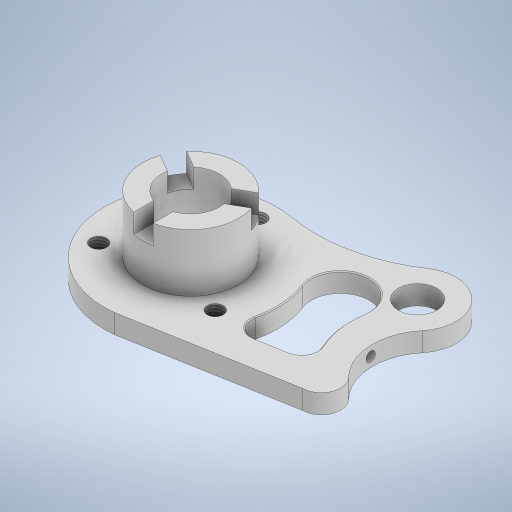
# Autodesk Inventor part: Curved disk example
Saved by Autodesk Inventor 2024 (Build 280153000, 153)
## iProperties
Created: 2023-05-09
Part Number: Curved disk example
Material: Generic
Document SubType Name: Modeling
Designer: Raj
Density: 1 g/cm^3
Appearance: Default
Author: Raj
Autodesk Inventor part; units mm, degrees
ref_plane "YZ Plane" through (0, 0, 0) normal (1, 0, 0) x (0, 1, 0)
ref_plane "XZ Plane" through (0, 0, 0) normal (0, 1, 0) x (-1, 0, 0)
sketch "Sketch1" plane through (0, 0, 0) normal (0, 0, 1) x (1, 0, 0)
  arc A0 (93.3944, 27.2324) -> (66.8467, 56.6014) centre (78, 40) ccw
  circle A1 centre (78, 40) radius 10
  arc A2 (88.012, -30) -> (95.1215, -12.9797) centre (88, -20) ccw
  arc A3 (93.3944, 27.2324) -> (95.1215, -12.9797) centre (116.4861, 8.081) ccw
  arc A4 (70.653, 19.7601) -> (41.8659, 16.5) centre (55.8211, 22) ccw
  line L0 (5.1648, -44.7026) -> (88.012, -30)
  line L1 (53.0014, -19.9632) -> (68.5014, -17.2125)
  arc A5 (70.653, 19.7601) -> (74.3556, -5.958) centre (115.1484, 13.0405) ccw
  arc A6 (43.8143, -10.2619) -> (53.0014, -19.9632) centre (51.6035, -12.0863) ccw
  arc A7 (68.5014, -17.2125) -> (74.3556, -5.958) centre (67.1035, -9.3356) ccw
  arc A8 (8.0041, 44.2824) -> (66.8467, 56.6014) centre (22.2337, 123.0068) ccw
  arc A9 (43.8143, -10.2619) -> (41.8659, 16.5) centre (0, 0) ccw
  arc A10 (8.0041, 44.2824) -> (5.1648, -44.7026) centre (0, 0) ccw
  dimension "d1" = 40
  dimension "d2" = 20
  dimension "d3" = 40
  dimension "d4" = 78
  dimension "d5" = 20
  dimension "d6" = 20
  dimension "d7" = 88
  dimension "d8" = 60
  dimension "d10" = 30
  dimension "d11" = 22
  dimension "d19" = 16
  dimension "d22" = 15.5
  dimension "d23" = 90
  dimension "d24" = 160
  dimension "d25" = 45
  dimension "d26" = 123.0068
  dimension "d27" = 44.9174
  dimension "d28" = 8
  dimension "d29" = 8
  dimension "d31" = 45
  dimension "d32" = 31.3356
  dimension "d33" = 34.0863
  dimension "d34" = 13.0404
  dimension "d70" = 55.8211
  constraints: 20 point on circle, 11 centre point, 6 tangent, 4 end point, 2 coincident, 1 parallel
  measures "d1" diameter of A0
  measures "d2" diameter of A1
  measures "d3" vertical distance of point (0, 0) A0.centre
  measures "d4" horizontal distance of point (0, 0) A0.centre
  measures "d5" diameter of A2
  measures "d6" vertical distance of A2.centre point (0, 0)
  measures "d7" horizontal distance of A2.centre point (0, 0)
  measures "d8" diameter of A3
  measures "d10" diameter of A4
  measures "d11" vertical distance of point (0, 0) A4.centre
  measures "d19" distance between parallel lines of L0 L1
  measures "d22" horizontal distance of A6.centre A7.centre
  measures "d23" diameter of A5
  measures "d24" diameter of A8
  measures "d25" radius of A10
  measures "d26" vertical distance of A9.centre A8.centre
  measures "d27" distance from line of A9.centre L0
  measures "d28" radius of A7
  measures "d29" radius of A6
  measures "d31" radius of A9
  measures "d32" vertical distance of A4.centre A7.centre
  measures "d33" vertical distance of A4.centre A6.centre
  measures "d34" vertical distance of A5.centre point (0, 0)
  measures "d70" horizontal distance of point (0, 0) A4.centre
extrude "Extrusion1" add sketch "Sketch1" along normal blind 10
sketch "Sketch2" plane through (0, 0, 10) normal (0, 0, 1) x (1, 0, 0)
  circle A0 centre (0, 0) radius 25
  circle A1 centre (0, 0) radius 15
  dimension "d37" = 50
  dimension "d38" = 30
  constraints: 2 centre point, 2 coincident
  measures "d37" diameter of A0
  measures "d38" diameter of A1
extrude "Extrusion2" add sketch "Sketch2" along normal blind 30
sketch "Sketch3" plane through (0, 0, 40) normal (0, 0, 1) x (1, 0, 0)
  line L0 (-5, -12.5) -> (5, -12.5)
  line L1 (5, -12.5) -> (5, -27.5)
  line L2 (5, -27.5) -> (-5, -27.5)
  line L3 (-5, -27.5) -> (-5, -12.5)
  line L4 (-5, -12.5) -> (5, -27.5) construction
  line L5 (5, -12.5) -> (-5, -27.5) construction
  line L6 (13.3253, 1.9199) -> (8.3253, 10.5801)
  line L7 (26.3157, 9.4199) -> (13.3253, 1.9199)
  line L8 (8.3253, 10.5801) -> (21.3157, 18.0801)
  line L9 (21.3157, 18.0801) -> (26.3157, 9.4199)
  line L10 (-8.3253, 10.5801) -> (-13.3253, 1.9199)
  line L11 (-21.3157, 18.0801) -> (-8.3253, 10.5801)
  line L12 (-13.3253, 1.9199) -> (-26.3157, 9.4199)
  line L13 (-26.3157, 9.4199) -> (-21.3157, 18.0801)
  point P0 (0, 0)
  point P1 (0, -20)
  dimension "d41" = 20
  dimension "d42" = 10
  dimension "d43" = 15
  dimension "d44" = 12.5
  dimension "d47" = 360
  constraints: 28 end point, 2 midpoint, 2 parallel, 1 horizontal, 1 perpendicular, 25 other
  measures "d41" distance of point (0, 0) point (0, -20)
  measures "d42" distance between parallel lines of L1 L3
  measures "d43" distance between parallel lines of L2 L0
  measures "d44" distance from line of point (0, 0) L0
extrude "Extrusion3" cut sketch "Sketch3" against normal blind 10
sketch "Sketch4" plane through (0, 0, 10) normal (0, 0, 1) x (1, 0, 0)
  point P0 (0, 0)
  point P1 (0, 35)
  dimension "d51" = 35
  measures "d51" distance of point (0, 35) point (0, 0)
hole "Hole1" at (0, 35, 10) direction (0, 0, -1) diameter 8.376 end through all thread size "M10x1.5" class "6H" standard "ISO Metric profile"
ref_plane "Work Plane1" through (70.1484, 13.0405, 0) normal (-1, 0, 0) x (0, 0, 1)
sketch "Sketch5" plane through (70.1484, 13.0405, 0) normal (-1, 0, 0) x (0, 0, 1)
  circle A0 centre (5, -6.0202) radius 2.5
  line L0 (0, 14.192) -> (0, -26.0202) projected
  line L1 (0, -26.0202) -> (10, -26.0202) projected
  point P0 (0, -13.0405)
  dimension "d59" = 5
  dimension "d60" = 5
  dimension "d61" = 20
  constraints: 1 centre point
  measures "d59" diameter of A0
  measures "d60" distance from line of L0 A0.centre
  measures "d61" distance from line of A0.centre L1
extrude "Extrusion4" cut sketch "Sketch5" against normal through all
pattern_circular "Circular Pattern1" count 3 over 360 about axis through (0, 0, 0) along (0, 0, 1) of "Hole1"
chamfer "Chamfer1" distance 0.5 angle 45 6 edges at (54.1332, 36.9047, 10) (70.6077, 6.628, 10) (74.2008, -13.0273, 10) (60.7514, -18.5878, 10) (45.7948, -17.5871, 10) (44.8812, 3.2676, 10)
body "Solid1"
